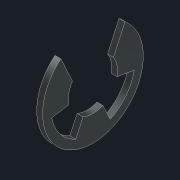
# Autodesk Inventor part: 10mm E-Clip
Saved by Autodesk Inventor 2022 (Build 260153000, 153)
## iProperties
Created: 2022-09-24
Part Number: 10mm E-Clip
Material: Steel, Wrought
Document SubType Name: Modeling
Designer: robpl
Density: 7.85 g/cm^3
Appearance: Iron Gray
Author: robpl
Autodesk Inventor part; units mm, degrees
ref_plane "YZ Plane" through (0, 0, 0) normal (1, 0, 0) x (0, 1, 0)
ref_plane "XZ Plane" through (0, 0, 0) normal (0, 1, 0) x (-1, 0, 0)
ref_plane "XY Plane" through (0, 0, 0) normal (0, 0, 1) x (1, 0, 0)
sketch "Sketch1" plane through (0, 0, 0) normal (1, 0, 0) x (0, 1, 0)
  circle A0 centre (0, 0) radius 10.2
  circle A1 centre (0, 0) radius 5
  circle A2 centre (0, 0) radius 8.5
  line L0 (7.8607, 6.5) -> (2.7739, 4.16)
  line L1 (2.7739, -4.16) -> (7.8607, -6.5)
  line L2 (-0.995, 4.9) -> (-1.5841, 8.3511)
  line L3 (-4.5826, 2) -> (-7.746, 3.5)
  line L4 (-4.5826, -2) -> (-7.746, -3.5)
  line L5 (-0.995, -4.9) -> (-1.5841, -8.3511)
  dimension "d0" = 20.4
  dimension "d1" = 10
  dimension "d2" = 8.32
  dimension "d4" = 17
  dimension "d5" = 13
  dimension "d6" = 4
  dimension "d7" = 7
  dimension "d8" = 9.8
  constraints: 12 end point, 12 point on circle, 5 vertical alignment, 4 equal length, 3 centre point, 3 coincident
  measures "d0" diameter of A0
  measures "d1" diameter of A1
  measures "d2" distance of L1.start L0.end
  measures "d4" diameter of A2
  measures "d5" distance of L1.end L0.start
  measures "d6" distance of L3.start L4.start
  measures "d7" distance of L4.end L3.end
  measures "d8" distance of L5.start L2.start
extrude "Extrusion1" add sketch "Sketch1" along normal blind 1.2 contours L0 A2 L1 A0 | L0 A1 L2 A2 | A2 L5 A1 L1 | L3 A1 L4 A2 picked at (4.4655, -8.4688)
body "Solid1"
